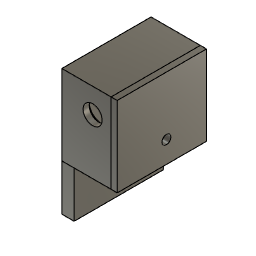
probe_jack_holder (Autodesk Fusion 360 design; units mm, degrees)
Autodesk Fusion 360 part; units mm, degrees
note: some values were not read from the file. Chosen so that the rebuilt part matches the saved one: which face or edge a step refers to. Set by a fixed rule: which sketch regions a step uses.
sketch "Sketch1" plane through (0, 0, 0) normal (0, 1, 0) x (1, 0, 0)
  circle A0 centre (0, 0) radius 3.1
  circle A1 centre (0, 0) radius 4.1
  line L0 (-3, -1) -> (-2.5, -1)
  line L1 (-2.5, -1) -> (-2.5, 1)
  line L2 (-2.5, 1) -> (-3, 1)
  line L3 (-3, 1) -> (-3, -1)
  line L4 (-1, -3) -> (1, -3)
  line L5 (1, -3) -> (1, -2.5)
  line L6 (1, -2.5) -> (-1, -2.5)
  line L7 (-1, -2.5) -> (-1, -3)
  line L8 (2.5, -1) -> (3, -1)
  line L9 (3, -1) -> (3, 1)
  line L10 (3, 1) -> (2.5, 1)
  line L11 (2.5, 1) -> (2.5, -1)
  dimension "d1" = 6.2
  dimension "d2" = 8.2
  constraint concentric A0 A1
  constraint horizontal L0
  constraint vertical L1
  constraint horizontal L2
  constraint vertical L3
  constraint horizontal L4
  constraint vertical L5
  constraint horizontal L6
  constraint vertical L7
  constraint horizontal L8
  constraint vertical L9
  constraint horizontal L10
  constraint vertical L11
  measures "d1" diameter of A0
  measures "d2" diameter of A1
extrude "Extrude1" add sketch "Sketch1" against normal blind 4 contours A0 L9 | A0 L8 L9 L10 L11 | A0 L0 L1 L2 L5 L6 L7 L8 L10 L11 | A0 L0 L1 L2 L3 | A0 L4 L5 L6 L7 | A0 L3 | A0 L4 makes body 1
extrude "Extrude2" add sketch "Sketch1" along normal blind 16 contours A0 L8 L9 L10 L11 | A0 L9 L10 | A0 L8 L9 | A0 L0 L1 L2 L3 | A0 L2 L3 | A0 L4 L5 | A0 L4 L5 L6 L7 | A0 L0 L3 | A0 L4 L7 bodies 1
extrude "Extrude3" add sketch "Sketch1" along normal blind 12 contours A0 L9 | A0 L0 L1 L2 L5 L6 L7 L8 L10 L11 | A0 L3 | A0 L4 | A1 bodies 1
ref_plane "WorkPlane1" through (-6, 0, 0) normal (1, 0, 0) x (0, 1, 0)
sketch "Sketch2" plane through (-6, 0, 0) normal (1, 0, 0) x (0, 1, 0)
  line L0 (-17, -13) -> (32, -13) construction
  line L1 (32, -13) -> (32, -33) construction
  line L2 (32, -33) -> (-17, -33) construction
  line L3 (-17, -33) -> (-17, -13) construction
  line L4 (-17, -26) -> (32, -26) construction
  line L5 (32, -26) -> (32, -20) construction
  line L6 (32, -20) -> (-17, -20) construction
  line L7 (-17, -20) -> (-17, -26) construction
  circle A0 centre (7, -23) radius 2.75
  line L8 (22, -20.5) -> (27, -20.5)
  line L9 (27, -20.5) -> (27, -25.5)
  line L10 (27, -25.5) -> (22, -25.5)
  line L11 (22, -25.5) -> (22, -20.5)
  line L12 (-2.4224, -33) -> (27, -33)
  line L13 (27, -33) -> (27, 5)
  line L14 (-2, 5) -> (-2, -9)
  line L15 (1, -4) -> (1, -9)
  line L16 (1, 4) -> (1, 5)
  line L17 (-2, 5) -> (-2, 8)
  line L18 (-2, 8) -> (27, 8)
  line L19 (27, 8) -> (27, 5)
  line L20 (1, 5) -> (24, 5)
  line L21 (24, 5) -> (24, -9)
  line L22 (-2, -9) -> (-2, -18)
  line L23 (-2, -18) -> (1, -18)
  line L24 (1, -18) -> (1, -9)
  line L25 (24, -9) -> (24, -33)
  circle A1 centre (7, -23) radius 5 construction
  line L26 (1, 4) -> (1, -4)
  circle A2 centre (14, -11) radius 3
  line L27 (-2, -18) -> (-2, -33)
  line L28 (27, -17) -> (24, -17)
  circle A3 centre (14, -11) radius 0.9
  dimension "d10" = 5.5
  dimension "d22" = 6
  dimension "d30" = 1.8
  constraint horizontal L0
  constraint vertical L1
  constraint horizontal L2
  constraint vertical L3
  constraint horizontal L4
  constraint vertical L5
  constraint horizontal L6
  constraint vertical L7
  constraint coincident L1 L5.end
  constraint coincident L3 L4.start
  constraint horizontal L8
  constraint vertical L9
  constraint horizontal L10
  constraint vertical L11
  constraint coincident L2 L12.start
  constraint coincident L2 L12.end
  constraint perpendicular L0 L13
  constraint vertical L14
  constraint vertical L15
  constraint vertical L16
  constraint parallel L14 L17
  constraint perpendicular L14 L18
  constraint perpendicular L18 L19
  constraint perpendicular L16 L20
  constraint perpendicular L20 L21
  constraint perpendicular L0 L22
  constraint perpendicular L22 L23
  constraint perpendicular L0 L24
  constraint coincident L2 L25.end
  constraint concentric A0 A1
  constraint parallel L15 L26
  constraint coincident L12 L27.end
  constraint coincident L13 L28.start
  constraint coincident L25 L28.end
  constraint perpendicular L25 L28
  constraint concentric A2 A3
  measures "d10" diameter of A0
  measures "d22" diameter of A2
  measures "d30" diameter of A3
extrude "Extrude4" add sketch "Sketch2" against normal blind 8 separate body contours L8 L10 L11 L25 | L8 L9 L10 L13 L25 makes body 2
extrude "Extrude5" add sketch "Sketch2" against normal blind 4 contours L8 L10 L11 L12 L15 L16 L20 L21 L23 L24 L25 L26 L27 | L8 L13 L25 L28 | L13 L14 L15 L16 L17 L18 L19 L20 L21 L22 L23 L24 L25 L26 L28 | L10 L12 L13 L25 | A2 bodies 2
extrude "Extrude6" add sketch "Sketch2" along normal blind 12 contours L13 L14 L15 L16 L17 L18 L19 L20 L21 L22 L23 L24 L25 L26 L28 | A2 bodies 2
sketch "Sketch3" plane through (0, -2, 0) normal (0, -1, 0) x (1, 0, 0)
  line L0 (6, 8) -> (-10, 8)
  line L1 (-10, 8) -> (-10, -18)
  line L2 (-6, -18) -> (6, -18)
  line L3 (6, -18) -> (6, 8)
  line L4 (-6, -33) -> (-6, 8)
  line L5 (6, 8) -> (6, -33)
  line L6 (6, -33) -> (-6, -33)
  circle A0 centre (0, -6) radius 2.5
  line L7 (-10, -18) -> (-6, -18)
  line L8 (-0.0955, -3.5018) -> (6, -3.5)
  line L9 (-0.0409, -8.4997) -> (6, -8.5)
  dimension "d23" = 5
  constraint coincident L0 L4.end
  constraint perpendicular L0 L4
  constraint coincident L0.start L3.end
  constraint perpendicular L0 L5
  constraint perpendicular L4 L6
  constraint coincident A0 L8.start
  constraint coincident L5 L8.end
  constraint coincident A0 L9.start
  constraint coincident L5 L9.end
  measures "d23" diameter of A0
extrude "Extrude11" cut sketch "Sketch3" along normal blind -29 and the other way blind 26 contours L3 L5 A0 L8 L9 bodies 2
combine "Combine2" operation cut target body 2 tool bodies 1 keep tools
sketch "Sketch4" plane through (6, 0, 0) normal (1, 0, 0) x (0, 1, 0)
  line L0 (24, -3.5) -> (27, -3.5)
  line L1 (27, -3.5) -> (27, 8)
  line L2 (27, 8) -> (-2, 8)
  line L3 (-2, 8) -> (-2, -18)
  line L4 (-2, -18) -> (1, -18)
  line L5 (1, -18) -> (1, 5)
  line L6 (1, 5) -> (24, 5)
  line L7 (24, 5) -> (24, -3.5)
  line L8 (-2, 8) -> (27, 8)
  line L9 (-2, 8) -> (-2, -33)
  line L10 (27, 8) -> (27, 5)
  line L11 (27, -33) -> (27, 5)
  line L12 (24, 5) -> (24, -9)
  line L13 (1, 5) -> (24, 5)
  line L14 (1, -18) -> (1, -9)
  line L15 (1, -4) -> (1, -9)
  line L16 (1, 4) -> (1, -4)
  line L17 (24, -9) -> (24, -33)
  circle A0 centre (14, -11) radius 0.9
  line L18 (1, -18) -> (27, -18)
  line L19 (1, -18) -> (-2, -18)
  line L20 (1, 5) -> (4, 5)
  line L21 (4, 5) -> (4, 2)
  line L22 (4, 2) -> (1, 2)
  line L23 (1, 2) -> (1, 5)
  line L24 (24, 5) -> (21, 5)
  line L25 (21, 5) -> (21, 2)
  line L26 (21, 2) -> (24, 2)
  line L27 (24, 2) -> (24, 5)
  circle A1 centre (14, -11) radius 1.25
  line L28 (24, -3.5) -> (27, -3.5)
  line L29 (27, -8.5) -> (24, -8.5)
  line L30 (24, -3.5) -> (22, -3.5)
  line L31 (22, -3.5) -> (22, -8.5)
  line L32 (22, -8.5) -> (24, -8.5)
  line L33 (24, -8.5) -> (24, -3.5)
  dimension "d35" = 3
  dimension "d36" = 3
  dimension "d37" = 3
  dimension "d38" = 3
  dimension "d39" = 2.5
  dimension "d44" = 2
  constraint coincident L4.end L5.start
  constraint coincident L11 L18.end
  constraint perpendicular L11 L18
  constraint coincident L3.end L4.start
  constraint horizontal L20
  constraint vertical L21
  constraint horizontal L22
  constraint vertical L23
  constraint coincident L5.end L6.start
  constraint horizontal L24
  constraint vertical L25
  constraint horizontal L26
  constraint vertical L27
  constraint coincident L6.end L7.start
  constraint concentric A0 A1
  constraint horizontal L30
  constraint vertical L31
  constraint horizontal L32
  constraint vertical L33
  constraint coincident L0.start L7.end
  measures "d35" distance of L5.end L20.end
  measures "d36" distance of L5.end L22.end
  measures "d37" distance of L6.end L24.end
  measures "d38" distance of L6.end L26.end
  measures "d39" diameter of A1
  measures "d44" distance of L0.start L30.end
extrude "Extrude12" add sketch "Sketch4" along normal blind 2 separate body contours L0 L1 L2 L3 L4 L5 L6 L7 L8 L9 L10 L11 L12 L13 L14 L15 L16 L19 L20 L23 L24 L27 L28 | L5 L6 L7 L12 L13 L14 L15 L16 L17 L18 L21 L22 L25 L26 L30 L31 L32 | L0 L11 L12 L28 L29 L33 | L12 L30 L31 L32 L33 | L6 L7 L12 L13 L24 L25 L26 L27 | L11 L12 L17 L18 L29 | L5 L6 L13 L16 L20 L21 L22 L23 makes body 3
extrude "Extrude13" add sketch "Sketch4" against normal blind 2 contours L5 L6 L13 L16 L20 L21 L22 L23 bodies 3
extrude "Extrude14" add sketch "Sketch4" against normal blind 6 contours L0 L11 L12 L28 L29 L33 | L12 L30 L31 L32 L33 bodies 3
move_face "OffsetFaces1" offset -0.2 4 faces at (4, 26, -8.5) (4, 23.6667, -3.5) (5.3333, 2, 5) (5.3333, 1, 3) on bodies 3
move_face "OffsetFaces2" offset -0.2 1 faces at (7.3333, 15.2438, -10.8755) on bodies 3
hidden bodies 1
named bodies: "jack", "probe_jack_holder", "probe_jack_top"
